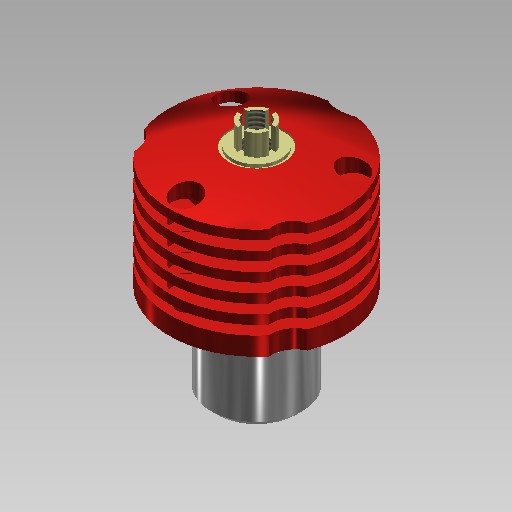
# Autodesk Inventor part: cylinder
Saved by Autodesk Inventor 2018.1 (Build 221171000, 171)
## iProperties
Created: 2013-08-26
Part Number: cylinder
Material: Generic
Document SubType Name: Modeling
Designer: Konstantin
Density: 1 g/cm^3
Appearance: Default
Mass: 8.02433 g
Surface Area: 84.6682 cm^2
Volume: 8.02433 cm^3
Author: Konstantin
Autodesk Inventor part; units mm, degrees
ref_plane "YZ Plane" through (0, 0, 0) normal (1, 0, 0) x (0, 1, 0)
sketch "Sketch1" plane through (0, 0, 0) normal (0, 0, 1) x (1, 0, 0)
  line L0 (9.5, 0) -> (14.25, 0)
  line L1 (14.25, 0) -> (14.25, 18)
  line L2 (0, -15) -> (7.5, -15)
  arc A0 (14.25, 18) -> (0, 20) centre (-0.9379, -38.4479) ccw
  line L3 (9.5, 0) -> (9.5, -3)
  line L4 (7.5, -3) -> (9.5, -3)
  line L5 (7.5, -3) -> (7.5, -15)
  line L6 (0, 20) -> (0, -15)
  constraints: 14 end point, 4 horizontal, 4 vertical, 3 perpendicular, 2 point on circle, 1 centre point, 1 parallel, 1 other
revolve "Revolution1" add sketch "Sketch1" angle 360 about axis through (0, 20, 0) along (0, -1, 0)
sketch "Sketch2" plane through (0, -15, 0) normal (0, -1, 0) x (1, 0, 0)
  circle A0 centre (0, 0) radius 6.5
  point P0 (0, 0)
  dimension "d8" = 13
  constraints: 1 centre point, 1 coincident
  measures "d8" diameter of A0
extrude "Extrusion1" cut sketch "Sketch2" against normal blind 24
ref_plane "Work Plane1" through (0, 20, 0) normal (0, 1, 0) x (-1, 0, 0)
sketch "Sketch3" plane through (0, 20, 0) normal (0, 1, 0) x (-1, 0, 0)
  circle A0 centre (0, 11.547) radius 2.25
  circle A1 centre (10, -5.7735) radius 2.25
  circle A2 centre (-10, -5.7735) radius 2.25
  constraints: 3 centre point, 3 other
sketch "Sketch4" plane through (0, 0, 0) normal (0, 0, 1) x (1, 0, 0)
  line L0 (8.75, 16.5) -> (18.9946, 16.5)
  line L1 (8.75, 15) -> (18.9946, 15)
  line L2 (8.75, 13.5) -> (18.9946, 13.5)
  line L3 (8.75, 12) -> (18.9946, 12)
  line L4 (8.75, 9) -> (18.9946, 9)
  line L5 (8.75, 10.5) -> (18.9946, 10.5)
  line L6 (8.75, 7.5) -> (18.9946, 7.5)
  line L7 (8.75, 6) -> (18.9946, 6)
  line L8 (8.75, 4.5) -> (18.9946, 4.5)
  line L9 (8.75, 3) -> (18.9946, 3)
  line L10 (0, 0) -> (0, 4.5) construction
  line L11 (18.9946, 16.5) -> (18.9946, 15)
  line L12 (8.75, 16.5) -> (8.75, 15)
  line L13 (18.9946, 13.5) -> (18.9946, 12)
  line L14 (18.9946, 10.5) -> (18.9946, 9)
  line L15 (18.9946, 7.5) -> (18.9946, 6)
  line L16 (18.9946, 4.5) -> (18.9946, 3)
  line L17 (8.75, 13.5) -> (8.75, 12)
  line L18 (8.75, 10.5) -> (8.75, 9)
  line L19 (8.75, 7.5) -> (8.75, 6)
  line L20 (8.75, 4.5) -> (8.75, 3)
  dimension "d27" = 0
  constraints: 42 end point, 11 vertical, 10 horizontal, 7 parallel
  measures "d27" distance from line of L10.end L8
revolve "Revolution2" cut sketch "Sketch4" angle 360 about axis through (0, 0, 0) along (0, 1, 0)
extrude "Extrusion2" cut sketch "Sketch3" against normal blind 16
sketch "Sketch5" plane through (0, 3, 0) normal (0, 1, 0) x (1, 0, 0)
  circle A0 centre (0, -11.547) radius 1.5
  circle A1 centre (10, 5.7735) radius 1.5
  circle A2 centre (-10, 5.7735) radius 1.5
  constraints: 3 centre point, 3 other
extrude "Extrusion3" cut sketch "Sketch5" against normal blind 5
sketch "Sketch6" plane through (0, 20, 0) normal (0, 1, 0) x (-1, 0, 0)
  circle A0 centre (0, -17.3205) radius 4
  circle A1 centre (15, 8.6603) radius 4
  circle A2 centre (-15, 8.6603) radius 4
  constraints: 3 centre point, 3 other
extrude "Extrusion4" cut sketch "Sketch6" against normal blind 25
sketch "Sketch7" plane through (0, 20, 0) normal (0, 1, 0) x (-1, 0, 0)
  circle A0 centre (0, 0) radius 4.5
  constraints: 1 centre point, 1 other
extrude "Extrusion5" cut sketch "Sketch7" against normal blind 0.5
sketch "Sketch8" plane through (0, 19.5, 0) normal (0, 1, 0) x (1, 0, 0)
  circle A0 centre (0, 0) radius 4
  dimension "d44" = 8
  constraints: 1 centre point, 1 coincident
  measures "d44" diameter of A0
extrude "Extrusion6" add sketch "Sketch8" along normal blind 0.5
sketch "Sketch9" plane through (0, 20, 0) normal (0, 1, 0) x (1, 0, 0)
  circle A0 centre (0, 0) radius 2.65
  constraints: 1 centre point, 1 other
extrude "Extrusion8" add sketch "Sketch9" along normal blind 3.5
sketch "Sketch10" plane through (0, 23.5, 0) normal (0, 1, 0) x (1, 0, 0)
  circle A0 centre (0, 0) radius 2
  constraints: 1 centre point, 1 coincident, 1 other
extrude "Extrusion9" cut sketch "Sketch10" against normal blind 12
thread "Thread1" size "M4x0.7" class "6H" standard "ISO Metric profile" full length
sketch "Sketch11" plane through (0, 23.5, 0) normal (0, 1, 0) x (1, 0, 0)
  arc A0 (0.5, 4.4721) -> (-0.5, 4.4721) centre (0, 0) ccw
  arc A1 (4.4721, -0.5) -> (4.4721, 0.5) centre (0, 0) ccw
  arc A2 (-4.4721, 0.5) -> (-4.4721, -0.5) centre (0, 0) ccw
  arc A3 (-0.5, -4.4721) -> (0.5, -4.4721) centre (0, 0) ccw
  line L0 (0.5, 4.4721) -> (0.5, 0.5)
  line L1 (0.5, -0.5) -> (0.5, -4.4721)
  line L2 (-4.4721, 0.5) -> (-0.5, 0.5)
  line L3 (0.5, 0.5) -> (4.4721, 0.5)
  line L4 (-0.5, 4.4721) -> (-0.5, 0.5)
  line L5 (-0.5, -0.5) -> (-0.5, -4.4721)
  line L6 (-4.4721, -0.5) -> (-0.5, -0.5)
  line L7 (0.5, -0.5) -> (4.4721, -0.5)
  constraints: 16 end point, 8 parallel, 8 point on circle, 4 centre point, 4 horizontal, 4 perpendicular, 4 vertical, 4 other
extrude "Extrusion10" cut sketch "Sketch11" against normal blind 3.5
ref_plane "Work Plane2" through (0, -1.5, 0) normal (0, -1, 0) x (1, 0, 0)
sketch "Sketch12" plane through (0, -1.5, 0) normal (0, -1, 0) x (1, 0, 0)
  line L0 (1.65, 10.1498) -> (1.65, 5.4417)
  line L1 (-1.65, 10.1498) -> (-1.65, 5.4417)
  line L2 (-9.615, -3.6459) -> (-5.5376, -1.2919)
  line L3 (-7.965, -6.5038) -> (-3.8876, -4.1498)
  line L4 (5.5376, -1.2919) -> (9.615, -3.6459)
  line L5 (3.8876, -4.1498) -> (7.965, -6.5038)
  arc A0 (5.5376, -1.2919) -> (1.65, 5.4417) centre (0, 0) ccw
  arc A1 (9.615, -3.6459) -> (1.65, 10.1498) centre (0, 0) ccw
  arc A2 (-1.65, 5.4417) -> (-5.5376, -1.2919) centre (0, 0) ccw
  arc A3 (-3.8876, -4.1498) -> (3.8876, -4.1498) centre (0, 0) ccw
  arc A4 (-1.65, 10.1498) -> (-9.615, -3.6459) centre (0, 0) ccw
  arc A5 (-7.965, -6.5038) -> (7.965, -6.5038) centre (0, 0) ccw
  point P0 (0, 0)
  constraints: 12 end point, 12 point on circle, 6 centre point, 2 parallel, 2 vertical, 10 other
extrude "Extrusion11" cut sketch "Sketch12" along normal mid plane 1.5
sketch "Sketch13" plane through (0, -3, 0) normal (0, -1, 0) x (1, 0, 0)
  line L0 (1.65, 8.096) -> (1.65, 5.5082)
  line L1 (-1.65, 5.5082) -> (-1.65, 8.096)
  line L2 (5.5952, -1.3251) -> (7.8363, -2.6191)
  line L3 (6.1863, -5.4769) -> (3.9452, -4.183)
  line L4 (-3.9452, -4.183) -> (-6.1863, -5.4769)
  line L5 (-7.8363, -2.6191) -> (-5.5952, -1.3251)
  arc A0 (7.8363, -2.6191) -> (1.65, 8.096) centre (0, 0) ccw
  arc A1 (5.5952, -1.3251) -> (1.65, 5.5082) centre (0, 0) ccw
  arc A2 (-1.65, 5.5082) -> (-5.5952, -1.3251) centre (0, 0) ccw
  arc A3 (-3.9452, -4.183) -> (3.9452, -4.183) centre (0, 0) ccw
  arc A4 (-1.65, 8.096) -> (-7.8363, -2.6191) centre (0, 0) ccw
  arc A5 (-6.1863, -5.4769) -> (6.1863, -5.4769) centre (0, 0) ccw
  constraints: 12 end point, 12 point on circle, 6 centre point, 2 vertical, 1 coincident, 10 other
extrude "Extrusion12" cut sketch "Sketch13" along normal blind 1.5
chamfer "Chamfer1" distance 1 angle 45 1 edges at (-7.5, -15, 0)
body "Solid1"
